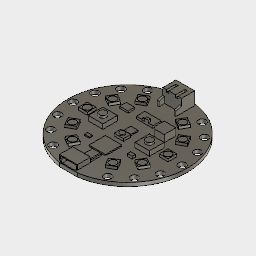
3333 Circuit Playground Express (Autodesk Fusion 360 design; units mm, degrees)
Autodesk Fusion 360 part; units mm, degrees
sketch "PCB" plane through (0, 0, 0) normal (0, 0, 1) x (1, 0, 0)
  circle A0 centre (0, 0) radius 25.43
  circle A1 centre (-23.1775, -0.0022) radius 1.6
  circle A2 centre (-21.779, -7.9292) radius 1.6
  circle A3 centre (-17.7536, -14.8999) radius 1.6
  circle A4 centre (-11.5868, -20.0734) radius 1.6
  circle A5 centre (11.5907, -20.0712) radius 1.6
  circle A6 centre (17.7564, -14.8965) radius 1.6
  circle A7 centre (21.7805, -7.9251) radius 1.6
  circle A8 centre (23.1775, 0.0022) radius 1.6
  circle A9 centre (21.779, 7.9292) radius 1.6
  circle A10 centre (17.7536, 14.8999) radius 1.6
  circle A11 centre (11.5868, 20.0734) radius 1.6
  circle A12 centre (-11.5907, 20.0712) radius 1.6
  circle A13 centre (-17.7564, 14.8965) radius 1.6
  circle A14 centre (-21.7805, 7.9251) radius 1.6
  circle A15 centre (-4.0226, -22.8258) radius 1.6
  circle A16 centre (4.0269, -22.825) radius 1.6
  circle A17 centre (4.0226, 22.8258) radius 1.6
  circle A18 centre (-4.0269, 22.825) radius 1.6
  line L0 (-10, -25.15) -> (10, -25.15)
  dimension "d1" = 50.86
  dimension "d6" = 3.2
  dimension "d8" = 360
  dimension "d160" = 25.15
  dimension "d168" = 23.1775
  measures "d1" diameter of A0
  measures "d6" diameter of A1
  measures "d160" distance of A0.centre L0
  measures "d168" distance of A0.centre A1.centre
extrude "Extrude1" add sketch "PCB" against normal blind 1.6 contours A0 L0 | A15 | A16 | A17 | A18 picked at (3.5956, 6.2293) makes body 1
sketch "microUSB" plane through (0, 0, 0) normal (0, 0, 1) x (1, 0, 0)
  line L0 (3.8, -25.15) -> (-3.8, -25.15)
  line L1 (-3.8, -25.15) -> (-3.8, -19.55)
  line L2 (-3.8, -19.55) -> (3.8, -19.55)
  line L3 (3.8, -19.55) -> (3.8, -25.15)
  line L4 (3.8, -25.15) -> (-3.8, -19.55) construction
  line L5 (-3.8, -25.15) -> (3.8, -19.55) construction
  line L6 (-3.7633, -25.15) -> (3.7633, -25.15)
  point P0 (0, -22.35)
  dimension "d156" = 7.6
  dimension "d157" = 5.6
  measures "d156" distance of L1.end L2.end
  measures "d157" distance of L0.end L1.end
extrude "Extrude2" add sketch "microUSB" along normal blind 3 separate body makes body 2
chamfer "Chamfer1" distance 1 angle 45 2 edges at (-3.8, -22.35, 0) (3.8, -22.35, 0) on bodies 2
shell "Shell3" thickness 0.4 removed faces 1 at (-0.9333, -25.15, 2) on bodies 2
sketch "JST base" plane through (0, 0, 0) normal (0, 0, 1) x (1, 0, 0)
  line L0 (4, 16.5) -> (-4, 16.5)
  line L1 (-4, 16.5) -> (-4, 24.5)
  line L2 (-4, 24.5) -> (4, 24.5)
  line L3 (4, 24.5) -> (4, 16.5)
  line L4 (4, 16.5) -> (-4, 24.5) construction
  line L5 (-4, 16.5) -> (4, 24.5) construction
  line L6 (0, 5) -> (0, -5)
  line L7 (-3.2, 16.5) -> (3.2, 16.5)
  line L8 (3.2, 16.5) -> (3.2, 18.9)
  line L9 (3.2, 18.9) -> (-3.2, 18.9)
  line L10 (-3.2, 18.9) -> (-3.2, 16.5)
  line L11 (-4, 18.9) -> (4, 18.9)
  point P0 (0, 20.5)
  dimension "d138" = 8
  dimension "d139" = 8
  dimension "d141" = 16.5
  dimension "d146" = 6.4
  dimension "d147" = 2.4
  dimension "d148" = 0.8
  measures "d138" distance of L1.end L2.end
  measures "d139" distance of L0.end L1.end
  measures "d141" distance of origin L0
  measures "d146" distance of L7.start L7.end
  measures "d147" distance of L7.start L9.end
  measures "d148" distance of L1 L10
extrude "Extrude3" add sketch "JST base" along normal blind 5.5 separate body contours L1 L2 L3 L9 L11 makes body 3
extrude "Extrude23" add sketch "JST base" along normal blind 2 contours L0 L3 L8 L11 | L0 L1 L10 L11 bodies 3
draft "Draft2" angle 15 neutral plane through (-3.2, 16.5, 0) pull (0, -1, 0) 1 faces at (-3.7333, 17.3, 2) on bodies 3
draft "Draft3" angle 15 neutral plane through (4, 16.5, 0) pull (0, -1, 0) 1 faces at (3.7333, 17.3, 2) on bodies 3
sketch "JST top" plane through (0, 0, 5.5) normal (0, 0, 1) x (-1, 0, 0)
  line L0 (-0.0003, -24.8336) -> (-0.0003, -18.8336) construction
  line L1 (2.4516, -22.8336) -> (1.4516, -22.8336)
  line L2 (1.4516, -22.8336) -> (1.4516, -18.8336)
  line L3 (1.4516, -18.8336) -> (2.4516, -18.8336)
  line L4 (2.4516, -18.8336) -> (2.4516, -22.8336)
  line L5 (-2.4521, -18.8336) -> (-2.4521, -22.8336)
  line L6 (-2.4521, -22.8336) -> (-1.4521, -22.8336)
  line L7 (-1.4521, -22.8336) -> (-1.4521, -18.8336)
  line L8 (-1.4521, -18.8336) -> (-2.4521, -18.8336)
  line L9 (0.5, -24.8336) -> (-0.5, -24.8336)
  line L10 (-0.5, -24.8336) -> (-0.5, -21)
  line L11 (-0.5, -21) -> (0.5, -21)
  line L12 (0.5, -21) -> (0.5, -24.8336)
  line L13 (4, -24.5) -> (4, -18.9)
  line L14 (4, -18.9) -> (-4, -18.9)
  line L15 (-4, -18.9) -> (-4, -24.5)
  line L16 (-4, -24.5) -> (4, -24.5)
  dimension "d18" = 1
  dimension "d19" = 4
  measures "d18" distance of L1.start L1.end
  measures "d19" distance of L1.start L3.end
sketch "JST hole" plane through (0, 24.5, 0) normal (0, 1, 0) x (-1, 0, 0)
  line L0 (4, 0) -> (4, 5.5)
  line L1 (4, 5.5) -> (-4, 5.5)
  line L2 (-4, 5.5) -> (-4, 0)
  line L3 (0.5, 5) -> (-0.5, 5)
  line L4 (-0.5, 5) -> (-0.5, 3)
  line L5 (-0.5, 3) -> (0.5, 3)
  line L6 (0.5, 3) -> (0.5, 5)
  line L7 (0.5, 5) -> (-0.5, 3) construction
  line L8 (-0.5, 5) -> (0.5, 3) construction
  line L9 (3, 4.5) -> (-3, 4.5)
  line L10 (-3, 4.5) -> (-3, 1)
  line L11 (-3, 1) -> (3, 1)
  line L12 (3, 1) -> (3, 4.5)
  line L13 (-4, 0) -> (4, 0)
  point P0 (0, 4)
extrude "Extrude4" cut sketch "JST top" against normal blind 1 contours L1 L2 L4 L14 | L2 L3 L4 L14 | L5 L7 L8 L14 | L5 L6 L7 L14 bodies 3
extrude "Extrude5" cut sketch "JST hole" against normal blind 5 contours L3 L4 L6 L9 | L4 L5 L6 L9 L10 L11 L12 | L4 L5 L6 L9 bodies 3
sketch "buttons" plane through (0, 0, 0) normal (0, 0, 1) x (1, 0, 0)
  line L0 (-6.806, -3.735) -> (-13.006, -3.735)
  line L1 (-13.006, -3.735) -> (-13.006, 2.465)
  line L2 (-13.006, 2.465) -> (-6.806, 2.465)
  line L3 (-6.806, 2.465) -> (-6.806, -3.735)
  line L4 (-6.806, -3.735) -> (-13.006, 2.465) construction
  line L5 (-13.006, -3.735) -> (-6.806, 2.465) construction
  circle A0 centre (-9.906, -0.635) radius 1.5
  point P0 (-9.906, -0.635)
  dimension "d162" = 6.2
  dimension "d163" = 6.2
  dimension "d164" = 9.906
  dimension "d166" = 3
  dimension "d169" = 0.635
  measures "d162" distance of L1.end L2.end
  measures "d163" distance of L0.end L1.end
  measures "d164" distance of origin A0.centre
  measures "d166" diameter of A0
  measures "d169" distance of origin A0.centre
extrude "Extrude6" add sketch "buttons" along normal blind 2 separate body contours L0 L1 L2 L3 | A0 makes body 4
extrude "Extrude7" add sketch "buttons" along normal blind 3 contours A0 bodies 4
mirror "Mirror2" about plane through (0, 0, 0) normal (1, 0, 0) of bodies 4 makes body 5
sketch "NeoPixels" plane through (0, 0, 0) normal (0, 0, 1) x (1, 0, 0)
  circle A0 centre (0, 0) radius 25.4
  line L0 (-15.295, -1.85) -> (-18.995, -1.85)
  line L1 (-18.995, -1.85) -> (-18.995, 1.85)
  line L2 (-18.995, 1.85) -> (-15.295, 1.85)
  line L3 (-15.295, 1.85) -> (-15.295, -1.85)
  line L4 (-15.295, -1.85) -> (-18.995, 1.85) construction
  line L5 (-18.995, -1.85) -> (-15.295, 1.85) construction
  circle A1 centre (-17.145, 0) radius 1.5
  line L6 (-18.995, 0) -> (-15.295, 0) construction
  line L7 (-17.3752, -7.8954) -> (-14.1709, -6.0454)
  circle A2 centre (-14.848, -8.5725) radius 1.5
  line L8 (-15.5252, -11.0996) -> (-17.3752, -7.8954)
  line L9 (-12.3209, -9.2496) -> (-15.5252, -11.0996)
  line L10 (-14.1709, -6.0454) -> (-12.3209, -9.2496)
  line L11 (-11.0996, -15.5252) -> (-9.2496, -12.3209)
  circle A3 centre (-8.5725, -14.848) radius 1.5
  line L12 (-7.8954, -17.3752) -> (-11.0996, -15.5252)
  line L13 (-6.0454, -14.1709) -> (-7.8954, -17.3752)
  line L14 (-9.2496, -12.3209) -> (-6.0454, -14.1709)
  line L15 (7.8954, -17.3752) -> (6.0454, -14.1709)
  circle A4 centre (8.5725, -14.848) radius 1.5
  line L16 (11.0996, -15.5252) -> (7.8954, -17.3752)
  line L17 (9.2496, -12.3209) -> (11.0996, -15.5252)
  line L18 (6.0454, -14.1709) -> (9.2496, -12.3209)
  line L19 (15.5252, -11.0996) -> (12.3209, -9.2496)
  circle A5 centre (14.848, -8.5725) radius 1.5
  line L20 (17.3752, -7.8954) -> (15.5252, -11.0996)
  line L21 (14.1709, -6.0454) -> (17.3752, -7.8954)
  line L22 (12.3209, -9.2496) -> (14.1709, -6.0454)
  line L23 (18.995, -1.85) -> (15.295, -1.85)
  circle A6 centre (17.145, 0) radius 1.5
  line L24 (18.995, 1.85) -> (18.995, -1.85)
  line L25 (15.295, 1.85) -> (18.995, 1.85)
  line L26 (15.295, -1.85) -> (15.295, 1.85)
  line L27 (17.3752, 7.8954) -> (14.1709, 6.0454)
  circle A7 centre (14.848, 8.5725) radius 1.5
  line L28 (15.5252, 11.0996) -> (17.3752, 7.8954)
  line L29 (12.3209, 9.2496) -> (15.5252, 11.0996)
  line L30 (14.1709, 6.0454) -> (12.3209, 9.2496)
  line L31 (11.0996, 15.5252) -> (9.2496, 12.3209)
  circle A8 centre (8.5725, 14.848) radius 1.5
  line L32 (7.8954, 17.3752) -> (11.0996, 15.5252)
  line L33 (6.0454, 14.1709) -> (7.8954, 17.3752)
  line L34 (9.2496, 12.3209) -> (6.0454, 14.1709)
  line L35 (-7.8954, 17.3752) -> (-6.0454, 14.1709)
  circle A9 centre (-8.5725, 14.848) radius 1.5
  line L36 (-11.0996, 15.5252) -> (-7.8954, 17.3752)
  line L37 (-9.2496, 12.3209) -> (-11.0996, 15.5252)
  line L38 (-6.0454, 14.1709) -> (-9.2496, 12.3209)
  line L39 (-15.5252, 11.0996) -> (-12.3209, 9.2496)
  circle A10 centre (-14.848, 8.5725) radius 1.5
  line L40 (-17.3752, 7.8954) -> (-15.5252, 11.0996)
  line L41 (-14.1709, 6.0454) -> (-17.3752, 7.8954)
  line L42 (-12.3209, 9.2496) -> (-14.1709, 6.0454)
  line L43 (-2.5, 0) -> (2.5, 0) construction
  line L44 (0, 2.5) -> (0, -2.5) construction
  point P0 (-17.145, 0)
  dimension "d40" = 50.8
  dimension "d41" = 3.7
  dimension "d42" = 3.7
  dimension "d43" = 3
  dimension "d46" = 360
  dimension "d131" = 17.145
  measures "d40" diameter of A0
  measures "d41" distance of L1.end L2.end
  measures "d42" distance of L0.end L1.end
  measures "d43" diameter of A1
  measures "d131" distance of P0 L44
extrude "Extrude8" add sketch "NeoPixels" along normal blind 1.1 separate body contours L0 L1 L2 L3 | A1 | L7 L8 L9 L10 | A2 | L11 L12 L13 L14 | A3 | L15 L16 L17 L18 | A4 | L19 L20 L21 L22 | A5 | L23 L24 L25 L26 | A6 | L27 L28 L29 L30 | A7 | L31 L32 L33 L34 | A8 | L35 L36 L37 L38 | A9 | L39 L40 L41 L42 | A10 makes body 6 at (8.7982, 14.0056, 0) makes body 7 at (8.3468, -15.6904, 0) makes body 8 at (-17.7617, 0.6167, 0) makes body 9 at (14.6223, -7.7301, 0) makes body 10 at (-8.3468, 15.6904, 0) makes body 11 at (15.6904, 8.3468, 0) makes body 12 at (-8.3468, -15.6904, 0) makes body 13 at (-15.6904, -8.3468, 0) makes body 14 at (16.5283, 0.6167, 0) makes body 15 at (-14.0056, 8.7982, 0)
extrude "Extrude9" cut sketch "NeoPixels" along normal blind 1.2 and the other way blind -1 contours A1 | A2 | A3 | A4 | A5 | A6 | A7 | A8 | A9 | A10 bodies 6 7 8 9 10 11 12 13 14 15
sketch "Switch" plane through (0, 0, 0) normal (0, 0, 1) x (1, 0, 0)
  line L0 (3.501, 7.242) -> (-3.499, 7.242)
  line L1 (-3.499, 7.242) -> (-3.499, 10.792)
  line L2 (-3.499, 10.792) -> (3.501, 10.792)
  line L3 (3.501, 10.792) -> (3.501, 7.242)
  line L4 (3.501, 7.242) -> (-3.499, 10.792) construction
  line L5 (-3.499, 7.242) -> (3.501, 10.792) construction
  line L6 (-1.5009, 8.242) -> (1.4991, 8.242)
  line L7 (1.4991, 8.242) -> (1.4991, 7.242)
  line L8 (1.4991, 7.242) -> (-1.5009, 7.242)
  line L9 (-1.5009, 7.242) -> (-1.5009, 8.242)
  line L10 (-0.0009, 7.242) -> (0.001, 10.792)
  line L11 (2.5, 0) -> (-2.5, 0) construction
  line L12 (0, -2.5) -> (0, 2.5) construction
  point P0 (0.001, 9.017)
  dimension "d53" = 7
  dimension "d54" = 3.55
  dimension "d55" = 3
  dimension "d56" = 1
  dimension "d104" = 9.017
  measures "d53" distance of L1.end L2.end
  measures "d54" distance of L0.end L1.end
  measures "d55" distance of L6.start L6.end
  measures "d56" distance of L6.start L8.end
  measures "d104" distance of P0 L11
extrude "Extrude10" add sketch "Switch" along normal blind 1 separate body makes body 16
extrude "Extrude12" cut sketch "Switch" along normal blind 1 and the other way blind -0.8 contours L0 L6 L7 L8 L10 | L0 L6 L8 L9 L10 bodies 16
extrude "Extrude11" add sketch "Switch" along normal blind 2 contours L0 L6 L7 L8 L10 bodies 16
sketch "buzzer" plane through (0, 0, 0) normal (0, 0, 1) x (1, 0, 0)
  line L0 (6.136, 9.358) -> (11.136, 9.358)
  line L1 (11.136, 9.358) -> (11.136, 4.358)
  line L2 (11.136, 4.358) -> (6.136, 4.358)
  line L3 (6.136, 4.358) -> (6.136, 9.358)
  line L4 (11.136, 4.358) -> (6.136, 9.358) construction
  line L5 (11.136, 9.358) -> (6.136, 4.358) construction
  line L6 (2.5, 0) -> (-2.5, 0) construction
  line L7 (0, -2.5) -> (0, 2.5) construction
  point P0 (8.636, 6.858)
  dimension "d64" = 5
  dimension "d65" = 5
  dimension "d99" = 6.858
  dimension "d100" = 8.636
  measures "d64" distance of L0.start L0.end
  measures "d65" distance of L0.start L2.end
  measures "d99" distance of L6 P0
  measures "d100" distance of L7 P0
extrude "Extrude13" add sketch "buzzer" along normal blind 3 separate body makes body 17
chamfer "Chamfer2" distance 1.1 angle 45 1 edges at (6.136, 4.358, 1.5) on bodies 17
sketch "mic" plane through (0, 0, 0) normal (0, 0, 1) x (1, 0, 0)
  line L0 (-3.499, 10.792) -> (-3.499, 7.242)
  line L1 (-3.499, 9.017) -> (-11.4283, 8.9278) construction
  line L2 (-7.364, 7.5535) -> (-10.924, 7.5535)
  line L3 (-10.924, 7.5535) -> (-10.924, 10.3535)
  line L4 (-10.924, 10.3535) -> (-7.364, 10.3535)
  line L5 (-7.364, 10.3535) -> (-7.364, 7.5535)
  line L6 (-7.364, 7.5535) -> (-10.924, 10.3535) construction
  line L7 (-10.924, 7.5535) -> (-7.364, 10.3535) construction
  line L8 (2.5, 0) -> (-2.5, 0) construction
  line L9 (0, -2.5) -> (0, 2.5) construction
  point P0 (-9.144, 8.9535)
  dimension "d74" = 2.8
  dimension "d75" = 3.56
  dimension "d106" = 9.144
  dimension "d107" = 8.9535
  measures "d74" distance of L2.end L3.end
  measures "d75" distance of L3.end L4.end
  measures "d106" distance of P0 L9
  measures "d107" distance of P0 L8
extrude "Extrude14" add sketch "mic" along normal blind 0.8 separate body makes body 18
sketch "reset btn" plane through (0, 0, 0) normal (0, 0, 1) x (1, 0, 0)
  line L0 (2.0015, -3.786) -> (-1.9985, -3.786)
  line L1 (-1.9985, -3.786) -> (-1.9985, -0.786)
  line L2 (-1.9985, -0.786) -> (2.0015, -0.786)
  line L3 (2.0015, -0.786) -> (2.0015, -3.786)
  line L4 (2.0015, -3.786) -> (-1.9985, -0.786) construction
  line L5 (-1.9985, -3.786) -> (2.0015, -0.786) construction
  line L6 (-2.5, 0) -> (2.5, 0) construction
  circle A0 centre (0.0015, -2.286) radius 1
  point P0 (0.0015, -2.286)
  dimension "d79" = 4
  dimension "d80" = 3
  dimension "d82" = 2
  dimension "d98" = 2.286
  measures "d79" distance of L1.end L2.end
  measures "d80" distance of L0.end L1.end
  measures "d82" diameter of A0
  measures "d98" distance of L6 P0
extrude "Extrude16" add sketch "reset btn" along normal blind 1 separate body contours L0 L1 L2 L3 | A0 makes body 19
extrude "Extrude17" add sketch "reset btn" along normal blind 0.5 from surface at 1 contours A0 bodies 19
sketch "light sensor" plane through (0, 0, 0) normal (0, 0, 1) x (1, 0, 0)
  line L0 (-2.5, 0) -> (2.5, 0) construction
  line L1 (0, 2.5) -> (0, -2.5) construction
  line L2 (10.3345, -8.447) -> (8.3345, -8.447)
  line L3 (8.3345, -8.447) -> (8.3345, -7.047)
  line L4 (8.3345, -7.047) -> (10.3345, -7.047)
  line L5 (10.3345, -7.047) -> (10.3345, -8.447)
  line L6 (10.3345, -8.447) -> (8.3345, -7.047) construction
  line L7 (8.3345, -8.447) -> (10.3345, -7.047) construction
  point P0 (9.3345, -7.747)
  dimension "d90" = 1.4
  dimension "d91" = 2
  dimension "d94" = 9.3345
  dimension "d95" = 7.747
  measures "d90" distance of L2.end L3.end
  measures "d91" distance of L3.end L4.end
  measures "d94" distance of L1 P0
  measures "d95" distance of L0 P0
extrude "Extrude18" add sketch "light sensor" along normal blind 1 separate body makes body 20
sketch "SAMD21" plane through (0, 0, 0) normal (0, 0, 1) x (1, 0, 0)
  line L0 (-3.5, -5.9615) -> (3.5, -5.9615)
  line L1 (3.5, -5.9615) -> (3.5, -12.9615)
  line L2 (3.5, -12.9615) -> (-3.5, -12.9615)
  line L3 (-3.5, -12.9615) -> (-3.5, -5.9615)
  line L4 (-3.5, -5.9615) -> (3.5, -12.9615) construction
  line L5 (3.5, -5.9615) -> (-3.5, -12.9615) construction
  line L6 (2.5, 0) -> (-2.5, 0) construction
  line L7 (0, 2.5) -> (0, -2.5) construction
  point P0 (0, -9.4615)
  dimension "d108" = 7
  dimension "d109" = 7
  dimension "d110" = 9.4615
  measures "d108" distance of L1.end L2.end
  measures "d109" distance of L0.end L1.end
  measures "d110" distance of P0 L6
extrude "Extrude19" add sketch "SAMD21" along normal blind 0.5 separate body makes body 21
sketch "SPI Flash" plane through (0, 0, 0) normal (0, 0, 1) x (1, 0, 0)
  line L0 (-1.2015, -13.6925) -> (2.5985, -13.6925)
  line L1 (2.5985, -13.6925) -> (2.5985, -18.6925)
  line L2 (2.5985, -18.6925) -> (-1.2015, -18.6925)
  line L3 (-1.2015, -18.6925) -> (-1.2015, -13.6925)
  line L4 (-1.2015, -13.6925) -> (2.5985, -18.6925) construction
  line L5 (2.5985, -13.6925) -> (-1.2015, -18.6925) construction
  line L6 (2.5, 0) -> (-2.5, 0) construction
  line L7 (0, -2.5) -> (0, 2.5) construction
  point P0 (0.6985, -16.1925)
  dimension "d113" = 3.8
  dimension "d114" = 5
  dimension "d115" = 0.6985
  dimension "d116" = 16.1925
  measures "d113" distance of L1.end L2.end
  measures "d114" distance of L0.end L1.end
  measures "d115" distance of P0 L7
  measures "d116" distance of P0 L6
extrude "Extrude20" add sketch "SPI Flash" along normal blind 1 separate body makes body 22
chamfer "Chamfer3" distance 0.3 angle 45 4 edges at (2.5985, -16.1925, 1) (0.6985, -18.6925, 1) (-1.2015, -16.1925, 1) (0.6985, -13.6925, 1) on bodies 22
sketch "accelerometer" plane through (0, 0, 0) normal (0, 0, 1) x (1, 0, 0)
  line L0 (-1.5, 2.897) -> (1.5, 2.897)
  line L1 (1.5, 2.897) -> (1.5, -0.103)
  line L2 (1.5, -0.103) -> (-1.5, -0.103)
  line L3 (-1.5, -0.103) -> (-1.5, 2.897)
  line L4 (-1.5, 2.897) -> (1.5, -0.103) construction
  line L5 (1.5, 2.897) -> (-1.5, -0.103) construction
  line L6 (2.5, 0) -> (-2.5, 0) construction
  point P0 (0, 1.397)
  dimension "d120" = 3
  dimension "d121" = 3
  dimension "d122" = 1.397
  measures "d120" distance of L0.end L1.end
  measures "d121" distance of L1.end L2.end
  measures "d122" distance of P0 L6
extrude "Extrude21" add sketch "accelerometer" along normal blind 0.5 separate body makes body 23
sketch "temp sensor" plane through (0, 0, 0) normal (0, 0, 1) x (1, 0, 0)
  line L0 (-8.366, -8.621) -> (-6.366, -8.621)
  line L1 (-6.366, -8.621) -> (-6.366, -9.921)
  line L2 (-6.366, -9.921) -> (-8.366, -9.921)
  line L3 (-8.366, -9.921) -> (-8.366, -8.621)
  line L4 (-8.366, -8.621) -> (-6.366, -9.921) construction
  line L5 (-6.366, -8.621) -> (-8.366, -9.921) construction
  line L6 (2.5, 0) -> (-2.5, 0) construction
  line L7 (0, -2.5) -> (0, 2.5) construction
  point P0 (-7.366, -9.271)
  dimension "d125" = 2
  dimension "d126" = 1.3
  dimension "d127" = 7.366
  dimension "d128" = 9.271
  measures "d125" distance of L1.end L2.end
  measures "d126" distance of L0.end L1.end
  measures "d127" distance of P0 L7
  measures "d128" distance of P0 L6
extrude "Extrude22" add sketch "temp sensor" along normal blind 0.5 separate body makes body 24
equation "d38 = 1 mm + 2 mm"
named bodies: "PCB", "microUSB", "JST", "left button", "neopixel 1", "neopixel 5", "neopixel 8", "neopixel 4", "neopixel 10", "neopixel 2", "neopixel 6", "neopixel 7", "neopixel 3", "neopixel 9", "on/off switch", "buzzer", "mic", "reset", "light sensor", "SAMD21", "SPI Flash", "accelerometer", "temp sensor", "right button"
